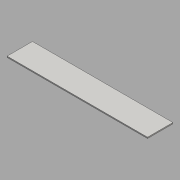
# Autodesk Inventor part: BASE LINEAR ACTUATOR
Saved by Autodesk Inventor 2016 (Build 200138000, 138)
## iProperties
Created: 2023-12-03
Part Number: BASE LINEAR ACTUATOR
Material: Generic
Document SubType Name: Modeling
Designer: Riskinova Oktavia
Density: 1 g/cm^3
Appearance: Default
Author: Riskinova Oktavia
Autodesk Inventor part; units mm, degrees
ref_plane "YZ Plane" through (0, 0, 0) normal (1, 0, 0) x (0, 1, 0)
ref_plane "XZ Plane" through (0, 0, 0) normal (0, 1, 0) x (-1, 0, 0)
ref_plane "XY Plane" through (0, 0, 0) normal (0, 0, 1) x (1, 0, 0)
sketch "Sketch1" plane through (0, 0, 0) normal (0, 0, 1) x (1, 0, 0)
  line L0 (-351.5, 63.5) -> (351.5, 63.5)
  line L1 (351.5, 63.5) -> (351.5, -63.5)
  line L2 (351.5, -63.5) -> (-351.5, -63.5)
  line L3 (-351.5, -63.5) -> (-351.5, 63.5)
  line L4 (-351.5, 63.5) -> (351.5, -63.5) construction
  line L5 (351.5, 63.5) -> (-351.5, -63.5) construction
  point P0 (0, 0)
  dimension "d0" = 703
  dimension "d1" = 127
  constraints: 12 end point, 2 midpoint, 2 parallel, 1 horizontal, 1 perpendicular
  measures "d0" distance of L0.start L0.end
  measures "d1" distance of L2.end L0.start
extrude "Extrusion1" add sketch "Sketch1" along normal mid plane 6
body "Solid1"
